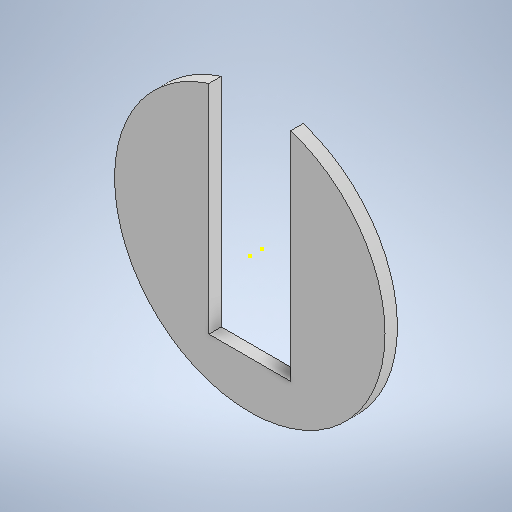
# Autodesk Inventor part: pomiedzy
Saved by Autodesk Inventor 2025 (Build 290162000, 162)
## iProperties
Created: 2024-04-17
Part Number: pomiedzy
Material: Generic
Document SubType Name: Modeling
Designer: bartek
Density: 1 g/cm^3
Appearance: Default
Author: bartek
Autodesk Inventor part; units mm, degrees
ref_plane "YZ Plane" through (0, 0, 0) normal (1, 0, 0) x (0, 1, 0)
ref_plane "XZ Plane" through (0, 0, 0) normal (0, 1, 0) x (-1, 0, 0)
ref_plane "XY Plane" through (0, 0, 0) normal (0, 0, 1) x (1, 0, 0)
sketch "Sketch1" plane through (0, 0, 0) normal (0, 0, 1) x (1, 0, 0)
  arc A0 (-5.75, 18.109) -> (5.75, 18.109) centre (0, 0) ccw
  line L0 (-5.75, -12.391) -> (5.75, -12.391)
  line L1 (-5.75, 18.109) -> (-5.75, -12.391)
  line L2 (5.75, -12.391) -> (5.75, 18.109)
  point P0 (0, -12.391)
  dimension "d0" = 38
  dimension "d1" = 11.5
  dimension "d2" = 30.5
  dimension "d3" = 30.5
  constraints: 6 end point, 2 midpoint, 2 point on circle, 2 vertical, 1 centre point, 1 coincident, 1 horizontal
  measures "d0" diameter of A0
  measures "d1" distance of L0.start L0.end
  measures "d2" distance of L1.start L0.start
  measures "d3" distance of L0.end L2.end
extrude "Extrusion1" add sketch "Sketch1" along normal blind 1.75
sketch "Sketch2" plane through (0, 0, 0) normal (0, 0, 1) x (1, 0, 0)
  point P0 (0, 0)
sketch "Sketch3" plane through (0, 0, 1.75) normal (0, 0, 1) x (1, 0, 0)
  point P0 (0, 0)
body "Solid1"
